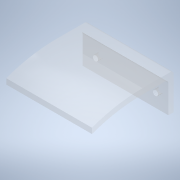
# Autodesk Inventor part: PolyWedge
Saved by Autodesk Inventor 2021 (Build 250183000, 183)
## iProperties
Created: 2021-05-22
Part Number: PolyWedge
Material: Polycarbonate, Clear
Document SubType Name: Modeling
Designer: sami8
Density: 1.2 g/cm^3
Appearance: Polycarbonate - Clear
Author: sami8
Autodesk Inventor part; units mm, degrees
ref_plane "YZ Plane" through (0, 0, 0) normal (1, 0, 0) x (0, 1, 0)
ref_plane "XZ Plane" through (0, 0, 0) normal (0, 1, 0) x (-1, 0, 0)
ref_plane "XY Plane" through (0, 0, 0) normal (0, 0, 1) x (1, 0, 0)
sketch "Sketch1" plane through (0, 0, 0) normal (1, 0, 0) x (0, 1, 0)
  line L0 (0, 0) -> (18, 0)
  line L1 (18, 0) -> (18, -3.175)
  line L2 (18, -3.175) -> (0, -3.175)
  line L3 (0, -3.175) -> (0, 0)
  line L4 (18, 0) -> (21.175, 0)
  line L5 (21.175, 0) -> (21.175, 15)
  line L6 (21.175, 15) -> (18, 15)
  line L7 (18, 15) -> (18, 0)
  line L8 (21.175, 0) -> (18, 0)
  line L9 (18, 0) -> (18, -3.175)
  line L10 (18, -3.175) -> (21.175, -3.175)
  line L11 (21.175, -3.175) -> (21.175, 0)
  arc A0 (21.175, 15) -> (15.9656, 44.5442) centre (-65.2066, 15) ccw
  line L12 (21.175, 15) -> (15.9656, 44.5442) construction
  line L13 (21.175, 15) -> (51.175, 15) construction
  line L14 (15.9656, 44.5442) -> (12.7906, 44.5442)
  arc A1 (18, 15) -> (12.7906, 44.5442) centre (-68.3816, 15) ccw
  line L15 (18, 15) -> (12.7906, 44.5442) construction
  line L16 (18, 15) -> (48, 15) construction
  dimension "d0" = 18
  dimension "d1" = 3.175
  dimension "d2" = 3.175
  dimension "d3" = 15
  dimension "d4" = 30
  dimension "d5" = 100
  dimension "d7" = 30
  dimension "d8" = 100
  constraints: 34 end point, 6 parallel, 5 horizontal, 4 point on circle, 3 perpendicular, 2 centre point, 2 equal length, 2 tangent
  measures "d0" distance of L1.end L2.end
  measures "d1" distance of L0.end L1.end
  measures "d2" distance of L6.end L5.end
  measures "d3" distance of L5.end L4.end
  measures "d4" distance of L5.end L12.end
  measures "d5" angle of L13 L12
  measures "d7" distance of L6.end L14.end
  measures "d8" angle of L16 L15
extrude "Extrusion1" add sketch "Sketch1" along normal mid plane 50
fillet "Fillet1" radius 2 2 edges at (0, 18, 0) (0, 21.175, -3.175)
sketch "Sketch2" plane through (25, 0, -3.175) normal (0, 0, -1) x (-1, 0, 0)
  line L0 (0, 0) -> (0, 19.175) projected
  line L1 (25, 0) -> (0, 0) projected
  line L2 (50, 19.175) -> (50, 0) projected
  line L3 (50, 7.5) -> (0, 7.5) construction
  circle A0 centre (7.5, 7.5) radius 1.55
  circle A1 centre (42.5, 7.5) radius 1.55
  dimension "d12" = 7.5
  dimension "d13" = 3.1
  dimension "d14" = 3.1
  dimension "d15" = 7.5
  dimension "d16" = 7.5
  constraints: 3 point on line, 2 centre point, 2 end point, 1 perpendicular, 2 other
  measures "d12" distance between parallel lines of L1 L3
  measures "d13" diameter of A0
  measures "d14" diameter of A1
  measures "d15" distance from line of L0 A0.centre
extrude "Extrusion2" cut sketch "Sketch2" against normal blind 10
body "Solid1"
